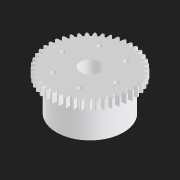
# Autodesk Inventor part: Spur Gear1
Saved by Autodesk Inventor 2017 SP1 (Build 210196100, 196)
## iProperties
Created: 2018-02-26
Part Number: Spur Gear1
Material: ABS Plastic
Document SubType Name: Modeling
Designer: Zach
Categories: <?xml version="1.0" encoding="UTF-16"?> <MemberInstance><Categories><FamilyTemplate><FamilyTemplateParameter ValueType="xs:double" Id="1" ObjectReferenceKey="da_z" ObjectType="kUserParameterObject"/><FamilyTemplateParameter ValueType="xs:double" Id="2" ObjectReferenceKey="da_b" ObjectType="kUserParameterObject"/><FamilyTemplateParameter ValueType="xs:double" Id="3" ObjectReferenceKey="da_beta" ObjectType="kUserParameterObject"/><FamilyTemplateParameter ValueType="xs:double" Id="4" ObjectReferenceKey="da_da" ObjectType="kUserParameterObject"/><FamilyTemplateParameter ValueType="xs:double" Id="5" ObjectReferenceKey="da_aw" ObjectType="kUserParameterObject"/><FamilyTemplateParameter ValueType="xs:string" Id="6" ObjectReferenceKey="EAIAABAAAACIAQAAAAAAAIAAAAAAAAAA" ObjectType="83910656" SubObjectId="SurfaceGeometry"/></FamilyTemplate><ParamToTemplateMap><ParamToTemplate CategoryParameter="//CategoryParameter[@InternalName='046C89C9-8512-4d59-83FE-43B91F4F132A']" TemplateParameter="1"/><ParamToTemplate CategoryParameter="//CategoryParameter[@InternalName='2552DF32-E462-4b46-AEBF-C6C7768E72AC']" TemplateParameter="2"/><ParamToTemplate CategoryParameter="//CategoryParameter[@InternalName='C9EE641D-15FC-4fae-A226-E94C4372FDD7']" TemplateParameter="3"/><ParamToTemplate><ParamToTemplate CategoryParameter="//CategoryParameter[@InternalName='00B6519A-459B-49c7-AD84-2E56D39A5744']" ConstantValue="0.000000"/></ParamToTemplate><ParamToTemplate><ParamToTemplate CategoryParameter="//CategoryParameter[@InternalName='04B31F0E-C7A6-4894-AA32-9629BEFACF47']" ConstantValue="1.000000"/></ParamToTemplate><ParamToTemplate><ParamToTemplate CategoryParameter="//CategoryParameter[@InternalName='43CBEC2E-7847-49e7-A936-2F7889FCB2D9']" ConstantValue="0.250000"/></ParamToTemplate><ParamToTemplate><ParamToTemplate CategoryParameter="//CategoryParameter[@InternalName='B1EFC894-105D-4ebd-86BF-FA20ED196853']" ConstantValue="0.350000"/></ParamToTemplate><ParamToTemplate><ParamToTemplate CategoryParameter="//CategoryParameter[@InternalName='51175063-3D10-4879-93E8-6246FE8B403D']" ConstantValue="2060000000.000000"/></ParamToTemplate><ParamToTemplate><ParamToTemplate CategoryParameter="//CategoryParameter[@InternalName='A3A52E27-4454-46a9-B0BD-C932399B70AF']" ConstantValue="0.300000"/></ParamToTemplate><ParamToTemplate><ParamToTemplate CategoryParameter="//CategoryParameter[@InternalName='91B76062-C214-41d9-B1B9-14D2AB99603D']" ConstantValue="0.200000"/></ParamToTemplate><ParamToTemplate><ParamToTemplate CategoryParameter="//CategoryParameter[@InternalName='374E806E-8B8A-4dda-A9AA-1039D6500AD2']" ConstantValue="5.000000"/></ParamToTemplate><ParamToTemplate><ParamToTemplate CategoryParameter="//CategoryParameter[@InternalName='2D373A89-B862-43d6-8D0B-0CBF12AB9F6C']" ConstantValue="0.392699"/></ParamToTemplate><ParamToTemplate CategoryParameter="//CategoryParameter[@InternalName='37777632-D6A2-4fac-9D53-DB8ACD95C989']" TemplateParameter="4"/><ParamToTemplate CategoryParameter="//CategoryParameter[@InternalName='FD1017F1-B727-4f7e-9707-0F86F1FF9423']" TemplateParameter="5"/><ParamToTemplate><ParamToTemplate CategoryParameter="//CategoryParameter[@InternalName='9E1B4470-B2D3-4ff1-B813-535BB4CDF51A']" ConstantValue="3520000.000000"/></ParamToTemplate><ParamToTemplate><ParamToTemplate CategoryParameter="//CategoryParameter[@InternalName='F8452263-BFF6-458c-9FB1-07C4B99E95CD']" ConstantValue="11400000.000000"/></ParamToTemplate><ParamToTemplate><ParamToTemplate CategoryParameter="//CategoryParameter[@InternalName='3E3BB259-FD49-497f-8171-6EBC954A3479']" ConstantValue="2.000000"/></ParamToTemplate><ParamToTemplate CategoryParameter="//CategoryParameter[@InternalName='27C3BAF2-7550-4e4b-AE2C-0DB134B7D9B7']" TemplateParameter="6"/></ParamToTemplateMap><Category DisplayName="Gear" InternalName="DC85795E-93AB-48d5-8EEE-5A27447B64BD" Mnemonic="Gear"><CategoryParameter DisplayName="z" InternalName="046C89C9-8512-4d59-83FE-43B91F4F132A" Mnemonic="z"/><CategoryParameter DisplayName="b" InternalName="2552DF32-E462-4b46-AEBF-C6C7768E72AC" Mnemonic="b"/><CategoryParameter DisplayName="||b|" InternalName="C9EE641D-15FC-4fae-A226-E94C4372FDD7" Mnemonic="beta"/><CategoryParameter DisplayName="x" InternalName="00B6519A-459B-49c7-AD84-2E56D39A5744" Mnemonic="x"/><CategoryParameter DisplayName="a*" InternalName="04B31F0E-C7A6-4894-AA32-9629BEFACF47" Mnemonic="a"/><CategoryParameter DisplayName="c*" InternalName="43CBEC2E-7847-49e7-A936-2F7889FCB2D9" Mnemonic="c"/><CategoryParameter DisplayName="r|.f|*" InternalName="B1EFC894-105D-4ebd-86BF-FA20ED196853" Mnemonic="rf"/><CategoryParameter DisplayName="E" InternalName="51175063-3D10-4879-93E8-6246FE8B403D" Mnemonic="E"/><CategoryParameter DisplayName="||m|" InternalName="A3A52E27-4454-46a9-B0BD-C932399B70AF" Mnemonic="mi"/><Category DisplayName="SpurGear" InternalName="26C5A22E-A91E-4dfd-A3B3-23CCAFAE1764" Mnemonic="SpurGear"><CategoryParameter DisplayName="m" InternalName="91B76062-C214-41d9-B1B9-14D2AB99603D" Mnemonic="m"/><CategoryParameter DisplayName="P" InternalName="374E806E-8B8A-4dda-A9AA-1039D6500AD2" Mnemonic="PP"/><CategoryParameter DisplayName="||a|" InternalName="2D373A89-B862-43d6-8D0B-0CBF12AB9F6C" Mnemonic="alpha"/><CategoryParameter DisplayName="d|.a|" InternalName="37777632-D6A2-4fac-9D53-DB8ACD95C989" Mnemonic="da"/><CategoryParameter DisplayName="a|.w|" InternalName="FD1017F1-B727-4f7e-9707-0F86F1FF9423" Mnemonic="aw"/><CategoryParameter DisplayName="||s||.Flim|" InternalName="9E1B4470-B2D3-4ff1-B813-535BB4CDF51A" Mnemonic="sFlim"/><CategoryParameter DisplayName="||s||.Hlim|" InternalName="F8452263-BFF6-458c-9FB1-07C4B99E95CD" Mnemonic="sHlim"/><CategoryParameter DisplayName="type" InternalName="3E3BB259-FD49-497f-8171-6EBC954A3479" Mnemonic="type"/><CategoryParameter DisplayName="PitchDiameter" InternalName="27C3BAF2-7550-4e4b-AE2C-0DB134B7D9B7" Mnemonic="IDS_PITCHDIAM"/></Category></Category></Categories></MemberInstance>
Density: 1.06 g/cm^3
Appearance: CR White
CustomPartVersion: 1
Author: Zach
Autodesk Inventor part; units mm, degrees
sketch "Sketch1" plane through (0, 0, 0) normal (0, 0, 1) x (1, 0, 0)
  circle A0 centre (0, 0) radius 47
  dimension "d0" = 94
  constraints: 1 centre point
  measures "d0" diameter of A0
extrude "Extrusion1" add sketch "Sketch1" along normal blind 4
ref_plane "Work Plane2" through (0, 0, 2) normal (0, 0, 1) x (1, 0, 0)
sketch "Sketch2" plane through (0, 0, 0) normal (0, 0, -1) x (-1, 0, 0)
  circle A0 centre (0, 0) radius 47 projected
  circle A1 centre (0, 0) radius 45
  dimension "d3" = 90
  constraints: 1 centre point, 1 coincident
  measures "d3" diameter of A1
surface extrude "Pitch Diameter" sketch "Sketch2" against normal through all shown no curves A1
ref_plane "Work Plane8" through (0, 0, 0) normal (0.9975641, 0.0697565, 0) x (0, 0, 1)
ref_plane "Work Plane9" through (0, 0, 0) normal (1, 0, 0) x (0, 1, 0)
spur gear teeth "Spur Gear" teeth 45 pitch diameter 90 tip diameter 94 root diameter 85 face width 4 start plane through (0, 0, 0) normal (0, 0, -1) x (-1, 0, 0)
sketch "Sketch3" plane through (0, 0, 0) normal (0, 0, -1) x (-1, 0, 0)
  circle A0 centre (0, 0) radius 37.5
  dimension "d49" = 75
  constraints: 1 centre point, 1 coincident
  measures "d49" diameter of A0
extrude "Extrusion2" add sketch "Sketch3" along normal blind 35
sketch "Sketch4" plane through (0, 0, -35) normal (0, 0, -1) x (-1, 0, 0)
  circle A0 centre (0, 0) radius 10.5
  dimension "d53" = 21
  constraints: 1 centre point, 1 coincident
  measures "d53" diameter of A0
extrude "Extrusion3" cut sketch "Sketch4" against normal blind 6
sketch "Sketch5" plane through (0, 0, -29) normal (0, 0, -1) x (-1, 0, 0)
  circle A0 centre (0, 0) radius 2.5
  circle A1 centre (-6.35, 0) radius 1.5
  circle A2 centre (0, -6.35) radius 1.5
  circle A3 centre (6.35, 0) radius 1.5
  circle A4 centre (0, 6.35) radius 1.5
  dimension "d56" = 5
  dimension "d57" = 3
  dimension "d58" = 6.35
  dimension "d61" = 360
  constraints: 5 centre point, 1 coincident, 1 horizontal alignment, 9 other
  measures "d56" diameter of A0
  measures "d57" diameter of A1
  measures "d58" distance of A1.centre point (0, 0)
extrude "Extrusion4" cut sketch "Sketch5" against normal through all
sketch "Sketch6" plane through (0, 0, 4) normal (0, 0, 1) x (1, 0, 0)
  circle A0 centre (30, 0) radius 2.5
  circle A1 centre (15, 25.9808) radius 2.5
  circle A2 centre (-15, 25.9808) radius 2.5
  circle A3 centre (-30, 0) radius 2.5
  circle A4 centre (-15, -25.9808) radius 2.5
  circle A5 centre (15, -25.9808) radius 2.5
  point P0 (0, 0)
  dimension "d65" = 5
  dimension "d66" = 30
  dimension "d69" = 360
  constraints: 6 centre point, 1 horizontal alignment, 13 other
  measures "d65" diameter of A0
  measures "d66" distance of A0.centre point (0, 0)
extrude "Extrusion5" cut sketch "Sketch6" against normal through all
sketch "Sketch7" plane through (0, 0, 4) normal (0, 0, 1) x (1, 0, 0)
  circle A0 centre (-15, -25.9808) radius 2.5 projected
  circle A1 centre (-15, 25.9808) radius 2.5 projected
  circle A2 centre (30, 0) radius 2.5 projected
  circle A3 centre (15, 25.9808) radius 2.5 projected
  circle A4 centre (-30, 0) radius 2.5 projected
  circle A5 centre (15, -25.9808) radius 2.5 projected
  circle A6 centre (0, 6.35) radius 1.5 projected
  circle A7 centre (0, -6.35) radius 1.5 projected
  circle A8 centre (6.35, 0) radius 1.5 projected
  circle A9 centre (-6.35, 0) radius 1.5 projected
  circle A10 centre (0, 0) radius 2.5 projected
  arc A11 (-7.3524, 46.4214) -> (-8.1094, 41.7192) centre (15.0688, 40.3999) ccw projected
  arc A12 (-8.1094, 41.7192) -> (-9.5604, 41.4107) centre (0, 0) ccw projected
  arc A13 (-9.5604, 41.4107) -> (-12.1645, 45.3985) centre (-30.1982, 30.7781) ccw projected
  arc A14 (-12.1645, 45.3985) -> (-13.7415, 44.9463) centre (0, 0) ccw projected
  arc A15 (-13.7415, 44.9463) -> (-13.8366, 40.1845) centre (9.2996, 42.1039) ccw projected
  arc A16 (-13.8366, 40.1845) -> (-15.2306, 39.6772) centre (0, 0) ccw projected
  arc A17 (-15.2306, 39.6772) -> (-18.3644, 43.2637) centre (-34.1878, 26.2758) ccw projected
  arc A18 (-18.3644, 43.2637) -> (-19.8631, 42.5965) centre (0, 0) ccw projected
  arc A19 (-19.8631, 42.5965) -> (-19.2946, 37.8678) centre (3.3493, 42.9884) ccw projected
  arc A20 (-19.2946, 37.8678) -> (-20.6044, 37.1713) centre (0, 0) ccw projected
  arc A21 (-20.6044, 37.1713) -> (-24.2068, 40.2869) centre (-37.512, 21.2621) ccw projected
  arc A22 (-24.2068, 40.2869) -> (-25.598, 39.4175) centre (0, 0) ccw projected
  arc A23 (-25.598, 39.4175) -> (-24.377, 34.814) centre (-2.6661, 43.0362) ccw projected
  arc A24 (-24.377, 34.814) -> (-25.5771, 33.942) centre (0, 0) ccw projected
  arc A25 (-25.5771, 33.942) -> (-29.5781, 36.5259) centre (-40.106, 15.8345) ccw projected
  arc A26 (-29.5781, 36.5259) -> (-30.8348, 35.4714) centre (0, 0) ccw projected
  arc A27 (-30.8348, 35.4714) -> (-28.9849, 31.0825) centre (-8.6296, 42.2463) ccw projected
  arc A28 (-28.9849, 31.0825) -> (-30.052, 30.052) centre (0, 0) ccw projected
  arc A29 (-30.052, 30.052) -> (-34.3736, 32.0539) centre (-41.9194, 10.0988) ccw projected
  arc A30 (-34.3736, 32.0539) -> (-35.4714, 30.8348) centre (0, 0) ccw projected
  arc A31 (-35.4714, 30.8348) -> (-33.0287, 26.7461) centre (-14.4252, 40.6342) ccw projected
  arc A32 (-33.0287, 26.7461) -> (-33.942, 25.5771) centre (0, 0) ccw projected
  arc A33 (-33.942, 25.5771) -> (-38.5001, 26.9581) centre (-42.917, 4.1664) ccw projected
  arc A34 (-38.5001, 26.9581) -> (-39.4175, 25.598) centre (0, 0) ccw projected
  arc A35 (-39.4175, 25.598) -> (-36.4296, 21.8891) centre (-19.94, 38.2311) ccw projected
  arc A36 (-36.4296, 21.8891) -> (-37.1713, 20.6044) centre (0, 0) ccw projected
  arc A37 (-37.1713, 20.6044) -> (-41.8773, 21.3376) centre (-43.0791, -1.847) ccw projected
  arc A38 (-41.8773, 21.3376) -> (-42.5965, 19.8631) centre (0, 0) ccw projected
  arc A39 (-42.5965, 19.8631) -> (-39.1215, 16.6061) centre (-25.0667, 35.084) ccw projected
  arc A40 (-39.1215, 16.6061) -> (-39.6772, 15.2306) centre (0, 0) ccw projected
  arc A41 (-39.6772, 15.2306) -> (-44.4394, 15.3017) centre (-42.4028, -7.8245) ccw projected
  arc A42 (-44.4394, 15.3017) -> (-44.9463, 13.7415) centre (0, 0) ccw projected
  arc A43 (-44.9463, 13.7415) -> (-41.0518, 10.9998) centre (-29.7055, 31.2539) ccw projected
  arc A44 (-41.0518, 10.9998) -> (-41.4107, 9.5604) centre (0, 0) ccw projected
  arc A45 (-41.4107, 9.5604) -> (-46.1365, 8.968) centre (-40.9012, -13.6497) ccw projected
  arc A46 (-46.1365, 8.968) -> (-46.4214, 7.3524) centre (0, 0) ccw projected
  arc A47 (-46.4214, 7.3524) -> (-42.1832, 5.1794) centre (-33.7661, 26.8156) ccw projected
  arc A48 (-42.1832, 5.1794) -> (-42.3383, 3.7041) centre (0, 0) ccw projected
  arc A49 (-42.3383, 3.7041) -> (-46.9356, 2.4598) centre (-38.6035, -19.2092) ccw projected
  arc A50 (-46.9356, 2.4598) -> (-46.9928, 0.8203) centre (0, 0) ccw projected
  arc A51 (-46.9928, 0.8203) -> (-42.4935, -0.7417) centre (-37.1695, 21.8553) ccw projected
  arc A52 (-42.4935, -0.7417) -> (-42.4418, -2.2243) centre (0, 0) ccw projected
  arc A53 (-42.4418, -2.2243) -> (-46.8212, -4.0963) centre (-35.5544, -24.3948) ccw projected
  arc A54 (-46.8212, -4.0963) -> (-46.6497, -5.7279) centre (0, 0) ccw projected
  arc A55 (-46.6497, -5.7279) -> (-41.9768, -6.6485) centre (-39.8494, 16.4696) ccw projected
  arc A56 (-41.9768, -6.6485) -> (-41.7192, -8.1094) centre (0, 0) ccw projected
  arc A57 (-41.7192, -8.1094) -> (-45.7954, -10.5727) centre (-31.8133, -29.1056) ccw projected
  arc A58 (-45.7954, -10.5727) -> (-45.3985, -12.1645) centre (0, 0) ccw projected
  arc A59 (-45.3985, -12.1645) -> (-40.643, -12.4258) centre (-41.7537, 10.7633) ccw projected
  arc A60 (-40.643, -12.4258) -> (-40.1845, -13.8366) centre (0, 0) ccw projected
  arc A61 (-40.1845, -13.8366) -> (-43.8783, -16.8433) centre (-27.453, -33.2499) ccw projected
  arc A62 (-43.8783, -16.8433) -> (-43.2637, -18.3644) centre (0, 0) ccw projected
  arc A63 (-43.2637, -18.3644) -> (-38.5181, -17.9613) centre (-42.8454, 4.8476) ccw projected
  arc A64 (-38.5181, -17.9613) -> (-37.8678, -19.2946) centre (0, 0) ccw projected
  arc A65 (-37.8678, -19.2946) -> (-41.1071, -22.7861) centre (-22.5583, -36.7471) ccw projected
  arc A66 (-41.1071, -22.7861) -> (-40.2869, -24.2068) centre (0, 0) ccw projected
  arc A67 (-40.2869, -24.2068) -> (-35.6435, -23.1472) centre (-43.103, -1.1625) ccw projected
  arc A68 (-35.6435, -23.1472) -> (-34.814, -24.377) centre (0, 0) ccw projected
  arc A69 (-34.814, -24.377) -> (-37.5359, -28.2853) centre (-17.2246, -39.529) ccw projected
  arc A70 (-37.5359, -28.2853) -> (-36.5259, -29.5781) centre (0, 0) ccw projected
  arc A71 (-36.5259, -29.5781) -> (-32.0752, -27.8825) centre (-42.5218, -7.15) ccw projected
  arc A72 (-32.0752, -27.8825) -> (-31.0825, -28.9849) centre (0, 0) ccw projected
  arc A73 (-31.0825, -28.9849) -> (-33.234, -33.234) centre (-11.5556, -41.5415) ccw projected
  arc A74 (-33.234, -33.234) -> (-32.0539, -34.3736) centre (0, 0) ccw projected
  arc A75 (-32.0539, -34.3736) -> (-27.8825, -32.0752) centre (-41.1129, -12.9983) ccw projected
  arc A76 (-27.8825, -32.0752) -> (-26.7461, -33.0287) centre (0, 0) ccw projected
  arc A77 (-26.7461, -33.0287) -> (-28.2853, -37.5359) centre (-5.6617, -42.7454) ccw projected
  arc A78 (-28.2853, -37.5359) -> (-26.9581, -38.5001) centre (0, 0) ccw projected
  arc A79 (-26.9581, -38.5001) -> (-23.1472, -35.6435) centre (-38.9038, -18.5936) ccw projected
  arc A80 (-23.1472, -35.6435) -> (-21.8891, -36.4296) centre (0, 0) ccw projected
  arc A81 (-21.8891, -36.4296) -> (-22.7861, -41.1071) centre (0.3425, -43.1174) ccw projected
  arc A82 (-22.7861, -41.1071) -> (-21.3376, -41.8773) centre (0, 0) ccw projected
  arc A83 (-21.3376, -41.8773) -> (-17.9613, -38.5181) centre (-35.9374, -23.827) ccw projected
  arc A84 (-17.9613, -38.5181) -> (-16.6061, -39.1215) centre (0, 0) ccw projected
  arc A85 (-16.6061, -39.1215) -> (-16.8433, -43.8783) centre (6.3399, -42.6501) ccw projected
  arc A86 (-16.8433, -43.8783) -> (-15.3017, -44.4394) centre (0, 0) ccw projected
  arc A87 (-15.3017, -44.4394) -> (-12.4258, -40.643) centre (-32.2716, -28.5967) ccw projected
  arc A88 (-12.4258, -40.643) -> (-10.9998, -41.0518) centre (0, 0) ccw projected
  arc A89 (-10.9998, -41.0518) -> (-10.5727, -45.7954) centre (12.2139, -41.3527) ccw projected
  arc A90 (-10.5727, -45.7954) -> (-8.968, -46.1365) centre (0, 0) ccw projected
  arc A91 (-8.968, -46.1365) -> (-6.6485, -41.9768) centre (-27.9776, -32.8097) ccw projected
  arc A92 (-6.6485, -41.9768) -> (-5.1794, -42.1832) centre (0, 0) ccw projected
  arc A93 (-5.1794, -42.1832) -> (-4.0963, -46.8212) centre (17.8503, -39.2504) ccw projected
  arc A94 (-4.0963, -46.8212) -> (-2.4598, -46.9356) centre (0, 0) ccw projected
  arc A95 (-2.4598, -46.9356) -> (-0.7417, -42.4935) centre (-23.1391, -36.3841) ccw projected
  arc A96 (-0.7417, -42.4935) -> (0.7417, -42.4935) centre (0, 0) ccw projected
  arc A97 (0.7417, -42.4935) -> (2.4598, -46.9356) centre (23.1391, -36.3841) ccw projected
  arc A98 (2.4598, -46.9356) -> (4.0963, -46.8212) centre (0, 0) ccw projected
  arc A99 (4.0963, -46.8212) -> (5.1794, -42.1832) centre (-17.8503, -39.2504) ccw projected
  arc A100 (5.1794, -42.1832) -> (6.6485, -41.9768) centre (0, 0) ccw projected
  arc A101 (6.6485, -41.9768) -> (8.968, -46.1365) centre (27.9776, -32.8097) ccw projected
  arc A102 (8.968, -46.1365) -> (10.5727, -45.7954) centre (0, 0) ccw projected
  arc A103 (10.5727, -45.7954) -> (10.9998, -41.0518) centre (-12.2139, -41.3527) ccw projected
  arc A104 (10.9998, -41.0518) -> (12.4258, -40.643) centre (0, 0) ccw projected
  arc A105 (12.4258, -40.643) -> (15.3017, -44.4394) centre (32.2716, -28.5967) ccw projected
  arc A106 (15.3017, -44.4394) -> (16.8433, -43.8783) centre (0, 0) ccw projected
  arc A107 (16.8433, -43.8783) -> (16.6061, -39.1215) centre (-6.3399, -42.6501) ccw projected
  arc A108 (16.6061, -39.1215) -> (17.9613, -38.5181) centre (0, 0) ccw projected
  arc A109 (17.9613, -38.5181) -> (21.3376, -41.8773) centre (35.9374, -23.827) ccw projected
  arc A110 (21.3376, -41.8773) -> (22.7861, -41.1071) centre (0, 0) ccw projected
  arc A111 (22.7861, -41.1071) -> (21.8891, -36.4296) centre (-0.3425, -43.1174) ccw projected
  arc A112 (21.8891, -36.4296) -> (23.1472, -35.6435) centre (0, 0) ccw projected
  arc A113 (23.1472, -35.6435) -> (26.9581, -38.5001) centre (38.9038, -18.5936) ccw projected
  arc A114 (26.9581, -38.5001) -> (28.2853, -37.5359) centre (0, 0) ccw projected
  arc A115 (28.2853, -37.5359) -> (26.7461, -33.0287) centre (5.6617, -42.7454) ccw projected
  arc A116 (26.7461, -33.0287) -> (27.8825, -32.0752) centre (0, 0) ccw projected
  arc A117 (27.8825, -32.0752) -> (32.0539, -34.3736) centre (41.1129, -12.9983) ccw projected
  arc A118 (32.0539, -34.3736) -> (33.234, -33.234) centre (0, 0) ccw projected
  arc A119 (33.234, -33.234) -> (31.0825, -28.9849) centre (11.5556, -41.5415) ccw projected
  arc A120 (31.0825, -28.9849) -> (32.0752, -27.8825) centre (0, 0) ccw projected
  arc A121 (32.0752, -27.8825) -> (36.5259, -29.5781) centre (42.5218, -7.15) ccw projected
  arc A122 (36.5259, -29.5781) -> (37.5359, -28.2853) centre (0, 0) ccw projected
  arc A123 (37.5359, -28.2853) -> (34.814, -24.377) centre (17.2246, -39.529) ccw projected
  arc A124 (34.814, -24.377) -> (35.6435, -23.1472) centre (0, 0) ccw projected
  arc A125 (35.6435, -23.1472) -> (40.2869, -24.2068) centre (43.103, -1.1625) ccw projected
  arc A126 (40.2869, -24.2068) -> (41.1071, -22.7861) centre (0, 0) ccw projected
  arc A127 (41.1071, -22.7861) -> (37.8678, -19.2946) centre (22.5583, -36.7471) ccw projected
  arc A128 (37.8678, -19.2946) -> (38.5181, -17.9613) centre (0, 0) ccw projected
  arc A129 (38.5181, -17.9613) -> (43.2637, -18.3644) centre (42.8454, 4.8476) ccw projected
  arc A130 (43.2637, -18.3644) -> (43.8783, -16.8433) centre (0, 0) ccw projected
  arc A131 (43.8783, -16.8433) -> (40.1845, -13.8366) centre (27.453, -33.2499) ccw projected
  arc A132 (40.1845, -13.8366) -> (40.643, -12.4258) centre (0, 0) ccw projected
  arc A133 (40.643, -12.4258) -> (45.3985, -12.1645) centre (41.7537, 10.7633) ccw projected
  arc A134 (45.3985, -12.1645) -> (45.7954, -10.5727) centre (0, 0) ccw projected
  arc A135 (45.7954, -10.5727) -> (41.7192, -8.1094) centre (31.8133, -29.1056) ccw projected
  arc A136 (41.7192, -8.1094) -> (41.9768, -6.6485) centre (0, 0) ccw projected
  arc A137 (41.9768, -6.6485) -> (46.6497, -5.7279) centre (39.8494, 16.4696) ccw projected
  arc A138 (46.6497, -5.7279) -> (46.8212, -4.0963) centre (0, 0) ccw projected
  arc A139 (46.8212, -4.0963) -> (42.4418, -2.2243) centre (35.5544, -24.3948) ccw projected
  arc A140 (42.4418, -2.2243) -> (42.4935, -0.7417) centre (0, 0) ccw projected
  arc A141 (42.4935, -0.7417) -> (46.9928, 0.8203) centre (37.1695, 21.8553) ccw projected
  arc A142 (46.9928, 0.8203) -> (46.9356, 2.4598) centre (0, 0) ccw projected
  arc A143 (46.9356, 2.4598) -> (42.3383, 3.7041) centre (38.6035, -19.2092) ccw projected
  arc A144 (42.3383, 3.7041) -> (42.1832, 5.1794) centre (0, 0) ccw projected
  arc A145 (42.1832, 5.1794) -> (46.4214, 7.3524) centre (33.7661, 26.8156) ccw projected
  arc A146 (46.4214, 7.3524) -> (46.1365, 8.968) centre (0, 0) ccw projected
  arc A147 (46.1365, 8.968) -> (41.4107, 9.5604) centre (40.9012, -13.6497) ccw projected
  arc A148 (41.4107, 9.5604) -> (41.0518, 10.9998) centre (0, 0) ccw projected
  arc A149 (41.0518, 10.9998) -> (44.9463, 13.7415) centre (29.7055, 31.2539) ccw projected
  arc A150 (44.9463, 13.7415) -> (44.4394, 15.3017) centre (0, 0) ccw projected
  arc A151 (44.4394, 15.3017) -> (39.6772, 15.2306) centre (42.4028, -7.8245) ccw projected
  arc A152 (39.6772, 15.2306) -> (39.1215, 16.6061) centre (0, 0) ccw projected
  arc A153 (39.1215, 16.6061) -> (42.5965, 19.8631) centre (25.0667, 35.084) ccw projected
  arc A154 (42.5965, 19.8631) -> (41.8773, 21.3376) centre (0, 0) ccw projected
  arc A155 (41.8773, 21.3376) -> (37.1713, 20.6044) centre (43.0791, -1.847) ccw projected
  arc A156 (37.1713, 20.6044) -> (36.4296, 21.8891) centre (0, 0) ccw projected
  arc A157 (36.4296, 21.8891) -> (39.4175, 25.598) centre (19.94, 38.2311) ccw projected
  arc A158 (39.4175, 25.598) -> (38.5001, 26.9581) centre (0, 0) ccw projected
  arc A159 (38.5001, 26.9581) -> (33.942, 25.5771) centre (42.917, 4.1664) ccw projected
  arc A160 (33.942, 25.5771) -> (33.0287, 26.7461) centre (0, 0) ccw projected
  arc A161 (33.0287, 26.7461) -> (35.4714, 30.8348) centre (14.4252, 40.6342) ccw projected
  arc A162 (35.4714, 30.8348) -> (34.3736, 32.0539) centre (0, 0) ccw projected
  arc A163 (34.3736, 32.0539) -> (30.052, 30.052) centre (41.9194, 10.0988) ccw projected
  arc A164 (30.052, 30.052) -> (28.9849, 31.0825) centre (0, 0) ccw projected
  arc A165 (28.9849, 31.0825) -> (30.8348, 35.4714) centre (8.6296, 42.2463) ccw projected
  arc A166 (30.8348, 35.4714) -> (29.5781, 36.5259) centre (0, 0) ccw projected
  arc A167 (29.5781, 36.5259) -> (25.5771, 33.942) centre (40.106, 15.8345) ccw projected
  arc A168 (25.5771, 33.942) -> (24.377, 34.814) centre (0, 0) ccw projected
  arc A169 (24.377, 34.814) -> (25.598, 39.4175) centre (2.6661, 43.0362) ccw projected
  arc A170 (25.598, 39.4175) -> (24.2068, 40.2869) centre (0, 0) ccw projected
  arc A171 (24.2068, 40.2869) -> (20.6044, 37.1713) centre (37.512, 21.2621) ccw projected
  arc A172 (20.6044, 37.1713) -> (19.2946, 37.8678) centre (0, 0) ccw projected
  arc A173 (19.2946, 37.8678) -> (19.8631, 42.5965) centre (-3.3493, 42.9884) ccw projected
  arc A174 (19.8631, 42.5965) -> (18.3644, 43.2637) centre (0, 0) ccw projected
  arc A175 (18.3644, 43.2637) -> (15.2306, 39.6772) centre (34.1878, 26.2758) ccw projected
  arc A176 (15.2306, 39.6772) -> (13.8366, 40.1845) centre (0, 0) ccw projected
  arc A177 (13.8366, 40.1845) -> (13.7415, 44.9463) centre (-9.2996, 42.1039) ccw projected
  arc A178 (13.7415, 44.9463) -> (12.1645, 45.3985) centre (0, 0) ccw projected
  arc A179 (12.1645, 45.3985) -> (9.5604, 41.4107) centre (30.1982, 30.7781) ccw projected
  arc A180 (9.5604, 41.4107) -> (8.1094, 41.7192) centre (0, 0) ccw projected
  arc A181 (8.1094, 41.7192) -> (7.3524, 46.4214) centre (-15.0688, 40.3999) ccw projected
  arc A182 (7.3524, 46.4214) -> (5.7279, 46.6497) centre (0, 0) ccw projected
  arc A183 (5.7279, 46.6497) -> (3.7041, 42.3383) centre (25.6208, 34.6814) ccw projected
  arc A184 (3.7041, 42.3383) -> (2.2243, 42.4418) centre (0, 0) ccw projected
  arc A185 (2.2243, 42.4418) -> (0.8203, 46.9928) centre (-20.5447, 37.9096) ccw projected
  arc A186 (0.8203, 46.9928) -> (-0.8203, 46.9928) centre (0, 0) ccw projected
  arc A187 (-0.8203, 46.9928) -> (-2.2243, 42.4418) centre (20.5447, 37.9096) ccw projected
  arc A188 (-2.2243, 42.4418) -> (-3.7041, 42.3383) centre (0, 0) ccw projected
  arc A189 (-3.7041, 42.3383) -> (-5.7279, 46.6497) centre (-25.6208, 34.6814) ccw projected
  arc A190 (-5.7279, 46.6497) -> (-7.3524, 46.4214) centre (0, 0) ccw projected
extrude "Extrusion6" add sketch "Sketch7" along normal blind 6
sketch "Sketch8" plane through (0, 0, 10) normal (0, 0, 1) x (1, 0, 0)
  circle A0 centre (0, 6.35) radius 1.5 projected
  circle A1 centre (0, -6.35) radius 1.5 projected
  circle A2 centre (6.35, 0) radius 1.5 projected
  circle A3 centre (-6.35, 0) radius 1.5 projected
  circle A4 centre (0, 0) radius 2.5 projected
  circle A5 centre (0, 0) radius 10.5 projected
extrude "Extrusion7" cut sketch "Sketch8" against normal blind 33 contours A0 | A1 | A2 | A3 | A4 | A5
equation "\"d0\" = da_da"
equation "\"d1\" = da_b"
equation "\"d3\" = da_dw"
equation "\"da_da\" = 94"
equation "\"da_b\" = 4"
equation "\"da_dw\" = 90"
body "Solid1"
body "Srf1"
